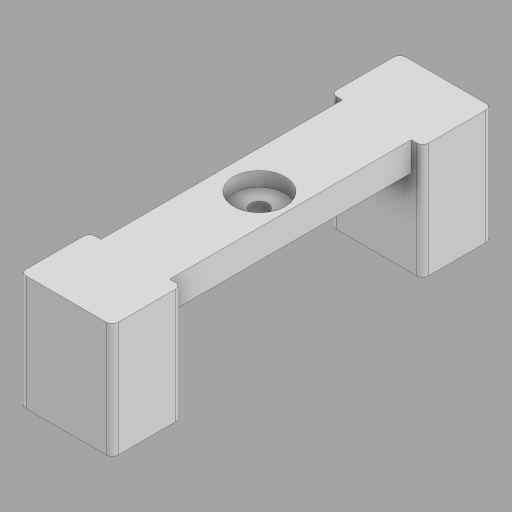
# Autodesk Inventor part: kick
Saved by Autodesk Inventor 2024.2 (Build 282272000, 272)
## iProperties
Created: 2024-01-02
Part Number: kick
Material: Типовые
Document SubType Name: Modeling
Designer: Fedor Orlov
Density: 1 g/cm^3
Appearance: По умолчанию
Author: Fedor Orlov
Autodesk Inventor part; units mm, degrees
ref_plane "YZ Plane" through (0, 0, 0) normal (1, 0, 0) x (0, 1, 0)
ref_plane "XZ Plane" through (0, 0, 0) normal (0, 1, 0) x (-1, 0, 0)
ref_plane "XY Plane" through (0, 0, 0) normal (0, 0, 1) x (1, 0, 0)
sketch "Эскиз1" plane through (0, 0, 0) normal (0, 1, 0) x (-1, 0, 0)
  line L0 (-6, -33) -> (6, -33)
  line L1 (6, -33) -> (6, 33)
  line L2 (6, 33) -> (-6, 33)
  line L3 (-6, 33) -> (-6, -33)
  line L4 (-6, -33) -> (6, 33) construction
  line L5 (6, -33) -> (-6, 33) construction
  circle A0 centre (-0.6, 0) radius 1.5
  point P0 (0, 0)
  dimension "d0" = 12
  dimension "d1" = 66
  dimension "d21" = 3
  dimension "d22" = 0.6
  dimension "d23" = 33
  constraints: 12 end point, 2 midpoint, 2 parallel, 1 centre point, 1 horizontal, 1 perpendicular
  measures "d0" distance of L2.end L1.end
  measures "d1" distance of L1.end L0.end
  measures "d21" diameter of A0
  measures "d22" distance of point (0, 0) A0.centre
  measures "d23" distance from line of L0 A0.centre
extrude "Выдавливание1" add sketch "Эскиз1" along normal blind 5
sketch "Эскиз2" plane through (0, 0, 0) normal (0, -1, 0) x (1, 0, 0)
  line L0 (-3, -33) -> (-8, -33)
  line L1 (-8, -33) -> (-8, -21)
  line L2 (-8, -21) -> (-3, -21)
  line L3 (-3, -21) -> (-3, -33) construction
  line L4 (-6, -33) -> (-6, 33) projected
  line L5 (6, -33) -> (-6, -33) projected
  line L6 (-6, 0) -> (6, 0) construction
  line L7 (6, 33) -> (6, -33) projected
  line L8 (0, -33) -> (0, 33) construction
  line L9 (-6, 33) -> (6, 33) projected
  line L10 (-3, 33) -> (-8, 33)
  line L11 (-8, 33) -> (-8, 21)
  line L12 (-8, 21) -> (-3, 21)
  line L13 (-3, 21) -> (-3, 33) construction
  line L14 (3, -33) -> (8, -33)
  line L15 (8, -33) -> (8, -21)
  line L16 (8, -21) -> (3, -21)
  line L17 (3, -21) -> (3, -33) construction
  line L18 (8, 21) -> (3, 21)
  line L19 (8, 33) -> (8, 21)
  line L20 (3, 33) -> (8, 33)
  line L21 (3, 21) -> (3, 33) construction
  line L22 (-3, -33) -> (3, -33)
  line L23 (-3, -21) -> (3, -21)
  line L24 (-3, 21) -> (3, 21)
  line L25 (-3, 33) -> (3, 33)
  point P0 (0, 0)
  dimension "d5" = 2
  dimension "d6" = 5
  dimension "d7" = 12
  dimension "d8" = 0
  constraints: 44 end point, 12 symmetric about line, 5 parallel, 4 midpoint, 1 collinear, 1 horizontal, 1 perpendicular
  measures "d5" distance between parallel lines of L1 L4
  measures "d6" distance between parallel lines of L3 L1
  measures "d7" distance between parallel lines of L0 L2
  measures "d8" distance between parallel lines of L5 L0
extrude "Выдавливание2" add sketch "Эскиз2" along normal blind 15 and the other way blind 5 contours L0 L4 L2 L23 L16 L7 L5 | L0 L1 L2 L4 | L7 L16 L15 L14 | L12 L11 L10 L4 | L4 L9 L7 L18 L24 L12 | L7 L20 L19 L18
fillet "Сопряжение1" radius 1 8 edges at (-8, -5, -21) (-8, -5, 33) (-8, -5, 21) (8, -5, -21) (8, -5, -33) (-8, -5, -33) (8, -5, 33) (8, -5, 21)
sketch "Эскиз3" plane through (0, 5, 0) normal (0, 1, 0) x (1, 0, 0)
  circle A0 centre (0.6, 0) radius 1.5 projected
  circle A1 centre (0.6, 0) radius 4.5
  point P0 (0, 0)
  dimension "d24" = 9
  constraints: 1 centre point, 1 coincident
  measures "d24" diameter of A1
extrude "Выдавливание3" cut sketch "Эскиз3" against normal blind 2.5
sketch "Эскиз4" plane through (0, -15, 0) normal (0, -1, 0) x (1, 0, 0)
  arc A0 (-7, -21) -> (-8, -22) centre (-7, -22) ccw projected
  arc A1 (7, -33) -> (8, -32) centre (7, -32) ccw projected
  line L0 (-7, -22) -> (7, -32) construction
  circle A2 centre (0, -27) radius 3
  line L1 (0, 0) -> (-6, 0) construction
  line L2 (-6, -21) -> (-6, 21) projected
  circle A3 centre (0, 27) radius 3
  dimension "d18" = 6
  constraints: 4 end point, 2 centre point, 2 midpoint, 1 symmetric about line, 1 other
  measures "d18" diameter of A2
extrude "Выдавливание4" cut sketch "Эскиз4" against normal blind 15
equation "\"d23\" = 0.5 * d1"
